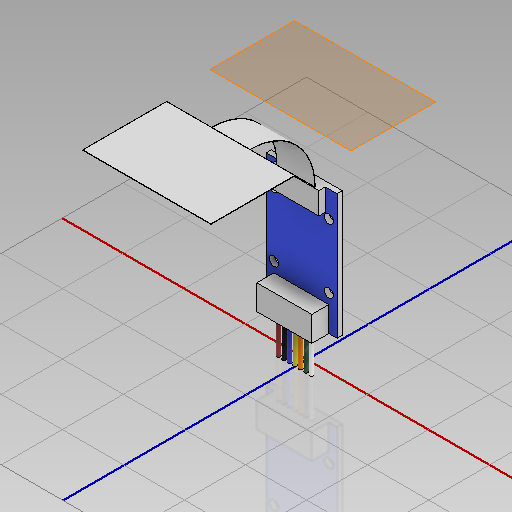
# Autodesk Inventor part: ЛЦМК000002.00.00.00.00.13 OLED
Saved by Autodesk Inventor 2021.2 (Build 252289000, 289)
## iProperties
Created: 2025-11-04
Part Number: ЛЦМК000002.00.00.00.00.13 OLED
Material: Типовые
Document SubType Name: Modeling
Designer: Захаров
Density: 1 g/cm^3
Appearance: По умолчанию
Author: Захаров
Autodesk Inventor part; units mm, degrees
ref_plane "YZ Plane" through (0, 0, 0) normal (1, 0, 0) x (0, 1, 0)
ref_plane "XZ Plane" through (0, 0, 0) normal (0, 1, 0) x (-1, 0, 0)
ref_plane "XY Plane" through (0, 0, 0) normal (0, 0, 1) x (1, 0, 0)
sketch "Эскиз1" plane through (0, 0, 0) normal (0, 0, 1) x (1, 0, 0)
  line L0 (-11.5, -21.5) -> (11.7, -21.5)
  line L1 (11.7, -21.5) -> (11.7, 19.5)
  line L2 (11.7, 19.5) -> (-11.5, 19.5)
  line L3 (-11.5, 19.5) -> (-11.5, -21.5)
  circle A0 centre (-9, -10.5) radius 1.5 projected
  point P0 (0, 0)
  dimension "d0" = 23.2
  dimension "d1" = 41
  dimension "d4" = 11
  dimension "d5" = 2.5
  constraints: 8 end point, 2 parallel, 1 horizontal, 1 perpendicular
  measures "d0" distance of L2.end L1.end
  measures "d1" distance of L1.end L0.end
  measures "d4" distance from line of L0 A0.centre
  measures "d5" distance from line of L3 A0.centre
extrude "Выдавливание1" add sketch "Эскиз1" along normal blind 1.7 contours L3 L2 L1 L0 | A0
sketch "Эскиз2" plane through (0, 0, 1.7) normal (0, 0, 1) x (1, 0, 0)
  circle A0 centre (-9, -9.9846) radius 1.5 projected
  circle A1 centre (9, -9.9846) radius 1.5 projected
  circle A2 centre (-9, 11.0154) radius 1.5 projected
  circle A3 centre (9, 11.0154) radius 1.5 projected
  point P0 (0, 0)
extrude "Выдавливание2" cut sketch "Эскиз2" against normal blind 1.7
sketch "Эскиз3" plane through (0, 0, 1.7) normal (0, 0, 1) x (1, 0, 0)
  line L0 (-9, -21.5) -> (9, -21.5)
  line L1 (9, -21.5) -> (9, -13.3)
  line L2 (9, -13.3) -> (-9, -13.3)
  line L3 (-9, -13.3) -> (-9, -21.5)
  line L4 (-11.5, -21.5) -> (11.7, -21.5) projected
  point P0 (0, 0)
  point P1 (0, -21.5)
  point P2 (0.1, -21.5)
  dimension "d8" = 18
  dimension "d9" = 8.2
  constraints: 8 end point, 2 midpoint, 2 parallel, 1 horizontal, 1 horizontal alignment, 1 perpendicular, 1 vertical alignment
  measures "d8" distance of L2.end L1.end
  measures "d9" distance of L1.end L0.end
extrude "Выдавливание3" add sketch "Эскиз3" along normal blind 5.6
sketch "Эскиз4" plane through (-11.5, -21.5, 0) normal (0, -1, 0) x (1, 0, 0)
  circle A0 centre (6, 3.65) radius 0.6
  line L0 (2.5, 7.3) -> (20.5, 7.3) projected
  line L1 (6, 7.3) -> (6, 0) construction
  line L2 (0, 0) -> (0, 1.7) projected
  circle A1 centre (7.8, 3.65) radius 0.6
  circle A2 centre (9.6, 3.65) radius 0.6
  circle A3 centre (11.4, 3.65) radius 0.6
  circle A4 centre (13.2, 3.65) radius 0.6
  circle A5 centre (15, 3.65) radius 0.6
  circle A6 centre (16.8, 3.65) radius 0.6
  point P0 (11.5, 0)
  dimension "d12" = 1.2
  dimension "d13" = 6
  dimension "d16" = 1.8
  constraints: 7 centre point, 2 end point, 1 coincident, 1 horizontal, 1 midpoint, 1 point on line, 1 vertical, 12 other
  measures "d12" diameter of A0
  measures "d13" distance from line of L2 A0.centre
  measures "d16" distance of A0.centre A1.centre
extrude "Выдавливание4" add sketch "Эскиз4" along normal blind 12.6
sketch "Эскиз5" plane through (0, 0, 1.7) normal (0, 0, 1) x (1, 0, 0)
  line L0 (-7.65, 12.3) -> (7.85, 12.3)
  line L1 (7.85, 12.3) -> (7.85, 19.5)
  line L2 (7.85, 19.5) -> (-7.65, 19.5)
  line L3 (-7.65, 19.5) -> (-7.65, 12.3)
  line L4 (11.7, 19.5) -> (-11.5, 19.5) projected
  point P0 (0, 0)
  point P1 (0.1, 19.5)
  point P2 (0.1, 19.5)
  dimension "d23" = 15.5
  dimension "d24" = 7.2
  constraints: 8 end point, 3 midpoint, 2 parallel, 1 coincident, 1 horizontal, 1 perpendicular
  measures "d23" distance of L2.end L1.end
  measures "d24" distance of L1.end L0.end
extrude "Выдавливание5" add sketch "Эскиз5" along normal blind 2.1
sketch "Эскиз6" plane through (-11.5, 19.5, 0) normal (0, 1, 0) x (1, 0, 0)
  line L0 (17.75, -3.5) -> (5.25, -3.5)
  line L1 (5.25, -3.5) -> (5.25, -3.4)
  line L2 (5.25, -3.4) -> (17.75, -3.4)
  line L3 (17.75, -3.4) -> (17.75, -3.5)
  line L4 (20.5, -7.3) -> (2.5, -7.3) projected
  line L5 (19.35, -3.8) -> (3.85, -3.8) projected
  point P0 (11.5, 0)
  point P1 (11.5, -3.4)
  point P2 (11.5, -7.3)
  dimension "d27" = 12.5
  dimension "d28" = 0.1
  dimension "d29" = 0.3
  constraints: 8 end point, 2 midpoint, 2 parallel, 1 horizontal, 1 perpendicular, 1 vertical alignment
  measures "d27" distance of L1.end L2.end
  measures "d28" distance of L0.end L1.end
  measures "d29" distance between parallel lines of L5 L0
sketch "Эскиз7" plane through (0, 0, 0) normal (1, 0, 0) x (0, 1, 0)
  line L0 (19.5, 3.4) -> (19.5, 3.5) projected
  line L1 (20.262, -17.8921) -> (54.1609, -17.8921) construction
  arc A0 (19.5, 3.5) -> (40.8268, 24.8268) centre (19.5, 24.8268) ccw
  line L2 (19.5, 1.7) -> (19.5, 3.8) projected
  line L3 (31.9208, 24.8268) -> (55.6437, 24.8268) construction
  point P0 (0, 0)
  dimension "d40" = 33.5
  constraints: 4 end point, 2 horizontal, 2 line through centre, 2 point on circle, 1 centre point, 1 point on line
sweep "Сдвиг1" add profiles "Эскиз6" path "Эскиз7" path curves A0
ref_plane "РабПлоскость2" through (0, 40.768, -17.8921) normal (0, 1, 0) x (-1, 0, 0)
sketch "Эскиз9" plane through (0, 40.768, -17.8921) normal (0, 1, 0) x (-1, 0, 0)
  line L0 (21, 70.2189) -> (-21, 70.2189)
  line L1 (-21, 70.2189) -> (-21, 42.7189)
  line L2 (-21, 42.7189) -> (21, 42.7189)
  line L3 (21, 42.7189) -> (21, 70.2189)
  line L4 (-6.25, 42.7189) -> (6.25, 42.7189) projected
  point P0 (0, 17.8921)
  point P1 (0, 42.7189)
  dimension "d41" = 42
  dimension "d42" = 27.5
  constraints: 8 end point, 2 midpoint, 2 parallel, 1 horizontal, 1 perpendicular
  measures "d41" distance of L2.end L1.end
  measures "d42" distance of L1.end L0.end
extrude "Выдавливание6" add sketch "Эскиз9" along normal blind 0.15
